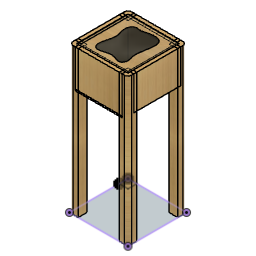
New let me fix it for you v6 (Autodesk Fusion 360 design; units mm, degrees)
Autodesk Fusion 360 part; units mm, degrees
ref_plane "Plan de construction1" through (0, 1000, 0) normal (0, 1, 0) x (0, 0, 1)
sketch "Esquisse1" plane through (0, 1000, 0) normal (0, 1, 0) x (1, 0, 0)
  line L0 (200, 200) -> (-200, 200)
  line L1 (-200, 200) -> (-200, -200)
  line L2 (-200, -200) -> (200, -200)
  line L3 (200, -200) -> (200, 200)
  line L4 (200, 200) -> (-200, -200) construction
  line L5 (-200, 200) -> (200, -200) construction
  dimension "d2" = 400
  constraint horizontal L0
  constraint perpendicular L0 L1
  constraint parallel L0 L2
  constraint parallel L1 L3
  constraint coincident L4 origin
  constraint coincident L5 origin
  constraint equal L0 L1
  measures "d2" distance of L0.start L0.end
sketch "Esquisse2" plane through (0, 0, 0) normal (0, 1, 0) x (1, 0, 0)
  line L0 (200, 200) -> (-200, 200)
  line L1 (-200, 200) -> (-200, -200)
  line L2 (-200, -200) -> (200, -200)
  line L3 (200, -200) -> (200, 200)
  line L4 (-200, 200) -> (-140, 200)
  line L5 (-140, 200) -> (-140, 140)
  line L6 (-140, 140) -> (-200, 140)
  line L7 (-200, 140) -> (-200, 200)
  dimension "d3" = 60
  constraint horizontal L4
  constraint vertical L5
  constraint horizontal L6
  constraint vertical L7
  constraint coincident L0 L1.start
  constraint coincident L1 L6.end
  constraint equal L5 L6
  measures "d3" distance of L5.end L6.end
extrude "Extrusion1" add sketch "Esquisse2" along normal up to surface (1000 mm away) contours L0 L1 L4 L5 L6 L7 makes body 1
fillet "Congé1" radius 25 1 edges at (-200, 500, -200) on bodies 1
pattern_circular "Réseau C1" count 4 over 360 about axis through (0, 1.75, 0) along (0, 1, 0) of bodies 1 makes body 2 at (-140, 333.3333, 160) makes body 3 at (160, 333.3333, 140) makes body 4 at (140, 333.3333, -160)
sketch "Esquisse6" plane through (0, 1000, 0) normal (0, 1, 0) x (1, 0, 0)
  line L0 (200, -160.0001) -> (160.0002, -160.0001)
  line L1 (160.0002, -160.0001) -> (160.0002, 160.0013)
  line L2 (160.0002, 160.0013) -> (200, 160.0013)
  line L3 (200, 160.0013) -> (200, -160.0001)
  line L4 (-160.0013, 200) -> (160.0001, 200)
  line L5 (160.0001, 160.0002) -> (-160.0013, 160.0002)
  line L6 (-160.0013, 160.0002) -> (-160.0013, 200)
  line L7 (160.0001, 200) -> (160.0001, 160.0002)
  line L8 (-200, -160.0013) -> (-200, 160.0001)
  line L9 (-160.0002, 160.0001) -> (-160.0002, -160.0013)
  line L10 (-160.0002, -160.0013) -> (-200, -160.0013)
  line L11 (-200, 160.0001) -> (-160.0002, 160.0001)
  line L12 (160.0013, -200) -> (-160.0001, -200)
  line L13 (-160.0001, -160.0002) -> (160.0013, -160.0002)
  line L14 (160.0013, -160.0002) -> (160.0013, -200)
  line L15 (-160.0001, -200) -> (-160.0001, -160.0002)
  dimension "d15" = 360
  constraint horizontal L0
  constraint vertical L1
  constraint horizontal L2
  constraint vertical L3
extrude "Extrusion2" add sketch "Esquisse6" against normal blind 230 separate body contours L0 L1 L2 L3 makes body 5
extrude "Extrusion3" add sketch "Esquisse6" against normal blind 250 separate body contours L12 L13 L14 L15 | L4 L5 L6 L7 | L8 L9 L10 L11 makes body 6 at (53.3342, 916.6667, 200) makes body 7 at (-160.0009, 916.6667, -53.333) makes body 8 at (53.333, 833.3333, -160.0009)
sketch "Esquisse15" plane through (0, 1000, 0) normal (0, 1, 0) x (1, 0, 0)
  line L0 (-175, 175) -> (175, 175)
  line L1 (175, 175) -> (175, -175)
  line L2 (175, -175) -> (-175, -175)
  line L3 (-175, -175) -> (-175, 175)
  constraint horizontal L0
  constraint vertical L1
  constraint horizontal L2
  constraint vertical L3
ref_plane "Plan de construction8" through (0, 750, 0) normal (0, 1, 0) x (1, 0, 0)
sketch "Esquisse17" plane through (0, 1000, 0) normal (0, 1, 0) x (1, 0, 0)
  line L0 (160, -200) -> (-160, -200)
  line L1 (-160, -200) -> (-160, 200)
  line L2 (-160, 200) -> (160, 200)
  line L3 (160, 200) -> (160, -200)
  constraint horizontal L0
  constraint vertical L1
  constraint horizontal L2
  constraint vertical L3
extrude "Extrusion9" add sketch "Esquisse17" against normal blind 10 from surface at -250 separate body makes body 9
extrude "Extrusion10" cut sketch "Esquisse15" against normal blind 3 bodies 1 2 3 4 5 6 7 8
extrude "Extrusion11" add sketch "Esquisse15" against normal blind 3 separate body makes body 10
ref_plane "Plan de construction9" through (0, 980, 0) normal (0, 1, 0) x (1, 0, 0)
extrude "Extrusion12" cut sketch "Esquisse15" along normal blind 3 from surface at -20 bodies 1 2 3 4 5 6 7 8
extrude "Extrusion13" add sketch "Esquisse15" along normal blind 3 from surface at -20 separate body makes body 11
sketch "Esquisse19" plane through (0, 1000, 0) normal (0, 1, 0) x (1, 0, 0)
  line L0 (107.45, 140.3) -> (-107.45, 140.3)
  line L1 (-107.45, 140.3) -> (-107.45, -140.3)
  line L2 (-107.45, -140.3) -> (107.45, -140.3)
  line L3 (107.45, -140.3) -> (107.45, 140.3)
  line L4 (107.45, 140.3) -> (-107.45, -140.3) construction
  line L5 (-107.45, 140.3) -> (107.45, -140.3) construction
  dimension "d66" = 214.9
  dimension "d67" = 280.6
  constraint horizontal L0
  constraint perpendicular L0 L1
  constraint parallel L0 L2
  constraint parallel L1 L3
  constraint coincident L4 origin
  constraint coincident L5 origin
  measures "d66" distance of L1.end L2.end
  measures "d67" distance of L0.end L1.end
extrude "Extrusion15" add sketch "Esquisse19" along normal blind 6.4 from surface at -17 bodies 11
ref_plane "Plan de construction10" through (0, 997, 0) normal (0, 1, 0) x (1, 0, 0)
extrude "Extrusion17" cut sketch "Esquisse15" against normal blind 3 from surface at -3 bodies 1 2 3 4 5 6 8 11
extrude "Extrusion18" add sketch "Esquisse15" against normal blind 3 from surface at -3 separate body makes body 12
sketch "Esquisse20" plane through (0, 1000, 0) normal (0, 1, 0) x (1, 0, 0)
  spline S0 degree 5 poles (2.9702, -120.1045) (7.0681, -119.8348) (15.2569, -119.7939) (27.4222, -121.4279) (43.0106, -127.0491) (61.2249, -134.4245) (77.5138, -136.2031) (91.0503, -127.6879) (98.8241, -110.0516) (98.8295, -90.0131) (94.6353, -72.3389) (90.1903, -60.1213) (88.8467, -53.3029) (88.4034, -45.7936) (88.4913, -33.5384) (89.8196, -15.0168) (93.0533, 9.1619) (97.7061, 35.6857) (101.4655, 59.537) (103.2857, 79.7063) (102.3989, 96.5235) (98.2065, 110.9745) (90.2444, 123.7985) (77.0958, 133.2881) (58.9031, 137.9279) (37.8289, 138.035) (16.5657, 134.6422) (-2.421, 129.4881) (-17.8557, 124.5172) (-30.8107, 121.6439) (-43.6339, 121.9352) (-58.1106, 124.5676) (-74.1441, 126.1002) (-87.4634, 118.7531) (-96.3647, 103.3877) (-100.3382, 83.9127) (-100.0369, 65.4428) (-96.4821, 49.6829) (-91.3708, 35.4015) (-86.8957, 21.1757) (-84.9832, 5.2069) (-86.8039, -13.7696) (-92.0527, -35.9447) (-98.6926, -60.0391) (-103.9624, -83.9818) (-105.043, -105.3549) (-100.0919, -121.9553) (-88.5831, -132.2499) (-73.2953, -136.0188) (-55.9982, -134.3536) (-37.333, -129.1226) (-21.5591, -124.2663) (-9.3306, -121.4124) (-1.1277, -120.3743) (2.9702, -120.1045) knots 0 0 0 0 0 0 0.02 0.04 0.06 0.08 0.1 0.12 0.14 0.16 0.18 0.2 0.22 0.24 0.26 0.28 0.3 0.32 0.34 0.36 0.38 0.4 0.42 0.44 0.46 0.48 0.5 0.52 0.54 0.56 0.58 0.6 0.62 0.64 0.66 0.68 0.7 0.72 0.74 0.76 0.78 0.8 0.82 0.84 0.86 0.88 0.9 0.92 0.94 0.96 0.98 1 1 1 1 1 1
  line L0 (-41.6235, -123.0399) -> (47.5639, -117.1691)
  line L1 (85.8055, -37.2443) -> (103.3819, 71.9806)
  line L2 (93.3383, -74.908) -> (85.8055, -37.2443)
  line L3 (71.5377, -150.9467) -> (110.117, -96.7951)
  line L4 (108.4038, 100.8562) -> (72.0487, 142.3216)
  line L5 (-102.9243, 107.4984) -> (-95.8249, 27.6746)
  line L6 (-30.9544, 124.4197) -> (-100, 125)
  line L7 (-111.5032, -112.7754) -> (-71.7545, -143.3305)
  point P0 (90.8274, -123.8709)
  point P1 (89.5719, -56.0761)
  point P2 (94.5937, 17.3682)
  point P3 (90.2262, 121.5889)
  point P4 (-5.2152, 128.4762)
  point P5 (-65.4772, 124.7099)
  point P6 (-99.3746, 67.5865)
  point P7 (-86.82, -8.9964)
  point P8 (-91.6288, -128.0529)
  constraint midpoint S0.start L0
  constraint midpoint P2 L1
  constraint midpoint P1 L2
  constraint coincident L1.start L2.end
  constraint midpoint P0 L3
  constraint midpoint P3 L4
  constraint midpoint P6 L5
  constraint midpoint P5 L6
  constraint midpoint P8 L7
extrude "Extrusion19" cut sketch "Esquisse20" against normal blind 3 from surface at -3 bodies 12
